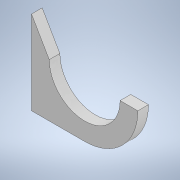
# Autodesk Inventor part: hook
Saved by Autodesk Inventor 2020.2 (Build 242310000, 310)
## iProperties
Created: 2020-03-15
Part Number: hook
Material: Generic
Document SubType Name: Modeling
Designer: robst
Density: 1 g/cm^3
Appearance: Default
Author: robst
Autodesk Inventor part; units mm, degrees
ref_plane "YZ Plane" through (0, 0, 0) normal (1, 0, 0) x (0, 1, 0)
ref_plane "XZ Plane" through (0, 0, 0) normal (0, 1, 0) x (-1, 0, 0)
ref_plane "XY Plane" through (0, 0, 0) normal (0, 0, 1) x (1, 0, 0)
sketch "Sketch1" plane through (0, 0, 0) normal (0, 0, 1) x (1, 0, 0)
  arc A0 (0, -19.05) -> (19.05, 0) centre (0, 0) ccw
  arc A1 (-12.7, 0) -> (12.7, 0) centre (0, 0) ccw
  line L0 (-19.05, 0) -> (19.05, 0) construction
  line L1 (-19.05, 0) -> (-19.05, -19.05)
  line L2 (-19.05, -19.05) -> (0, -19.05)
  line L3 (-19.05, 0) -> (-12.7, 0)
  line L4 (12.7, 0) -> (19.05, 0)
  circle A2 centre (0, 0) radius 19.05 construction
  dimension "d0" = 38.1
  dimension "d1" = 25.4
  constraints: 10 end point, 4 point on circle, 3 coincident, 2 centre point, 2 collinear, 2 point on line, 1 horizontal, 1 vertical, 1 vertical alignment, 2 other
  measures "d0" diameter of A0
  measures "d1" diameter of A1
extrude "Extrusion1" add sketch "Sketch1" along normal mid plane 3.81
sketch "Sketch2" plane through (0, 0, 0) normal (0, 0, 1) x (1, 0, 0)
  line L0 (-19.05, 0) -> (-12.7, 0) projected
  line L1 (-19.05, -19.05) -> (-19.05, 0) projected
  line L2 (-19.05, 0) -> (-19.05, 10.9985)
  line L3 (-19.05, 10.9985) -> (-12.7, 0)
  line L4 (-12.7, 0) -> (-19.05, 0)
  point P0 (0, 0)
  dimension "d5" = 60
  constraints: 6 end point, 1 collinear, 1 vertical
  measures "d5" angle of L0 L3
extrude "Extrusion2" add sketch "Sketch2" along normal mid plane 3.81
body "Solid1"
